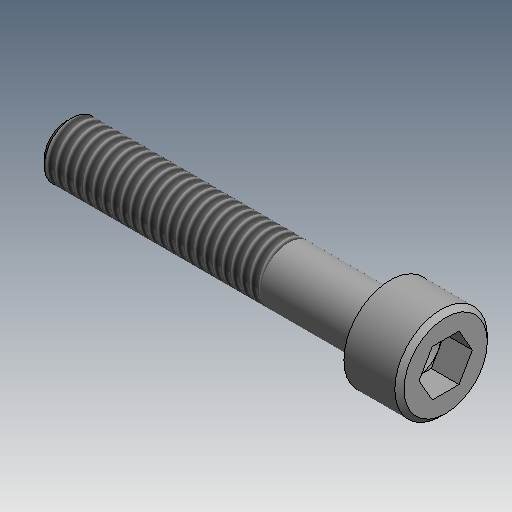
# Autodesk Inventor part: CBM6-35
Saved by Autodesk Inventor 2020 (Build 240168000, 168)
## iProperties
Part Number: CBM6-35
Material: 一般
Catalog Web Link: www.cadenas.de
Description: CBM-Hex Socket Head Cap Screws - Bright Chromate Plating
Vendor: MISUMI
Document SubType Name: Modeling
Designer: partserver
Manufacturer: MISUMI
Mass: 1.3796 g
Surface Area: 10.4152 cm^2
Volume: 1.3796 cm^3
Density: 1 g/cm^3
Appearance: PSOLRGB-192-192-192
Category: PARTsolutions
Company: MISUMI
PSOL_IDENT_0: {$CADENAS_DATA\23d-libs\misumi\metric\27_screws_nuts\cbm.prj},153 {VTYP=3D},{NB=CBM6-35},{LINA=CBM6-
PSOL_IDENT_1: 35},{NN=CBM},{DATE=07.06.2021 12:24:55},{GEOMDATE=24.03.2015 11:44:00},{VERSION=},{LINEID=30},{WBVAR=
PSOL_IDENT_2: L},{WBNUMERIC=L}  {NB=CBM6-35},{LINA=CBM6-35},{KT=DUMMY},{PN=CBM6-35},{TYPE=CBM},{M=6},{M1=6},{L=35}
PSOL_IDENT_3: ,{LALG=8,10,12,14,15,16,18,20,22,25,30,35,40,45,50,60},{LL=24},{A=10.0},{E=6},{B=5.0},{LL3D=24},{TT3
PSOL_IDENT_4: D=3},{R3D=0.250},{C3D=0.5},{A3D=-45}
NB: CBM6-35
NN: CBM
NT: Hex Socket Head Cap Screws - Bright Chromate Plating
NBSYN: $PN.
LINA: CBM6-35
CATALOG: Misumi
PN: CBM6-35
M: 6
L: 35
LL: 24
A: 10
E: 6
B: 5
SUPPLIER: MISUMI
ARTICLENO: CBM6-35
BOMINFO: CBM6-35
CREATOR: CADENAS GmbH
d12: 0.000 mm
d13: 0.000 mm
Title: CBM6-35
Author: Cadenas PARTsolutions
Comments: Hex Socket Head Cap Screws - Bright Chromate Plating
Autodesk Inventor part; units mm, degrees
sketch "Sketch_8" plane through (0, 0, 0) normal (0, 0, 1) x (1, 0, 0)
  line L0 (35, 0) -> (-6, 0)
  line L1 (-6, 0) -> (-6, 4.5)
  line L2 (-6, 4.5) -> (-5.5, 5)
  line L3 (-5.5, 5) -> (0, 5)
  line L4 (0, 5) -> (0, 3.25)
  arc A0 (0, 3.25) -> (0.25, 3) centre (0.25, 3.25) ccw
  line L5 (0.25, 3) -> (34.3865, 3)
  line L6 (34.3865, 3) -> (35, 2.3865)
  line L7 (35, 2.3865) -> (35, 0)
  line L8 (35, 0) -> (-6, 0)
  constraints: 18 end point, 2 point on circle, 1 centre point
revolve "Revolution1" add sketch "Sketch_8" angle 360 about axis through (35, 0, 0) along (1, 0, 0)
thread "Thread1" size "M6x1" class "6g" standard "ISO Metric profile" length 23.3865
sketch "Sketch2" plane through (-6, 0, 0) normal (-1, 0, 0) x (0, 0, 1)
  point P0 (0, 0)
hole "Hole1" at (-6, 0, 0) direction (1, 0, 0) diameter 5 depth 3 tip angle 120
sketch "Sketch_3" plane through (-6, 0, 0) normal (1, 0, 0) x (0, 0, -1)
  line L0 (-2.5, -1.4434) -> (0, -2.8868)
  line L1 (0, -2.8868) -> (2.5, -1.4434)
  line L2 (2.5, -1.4434) -> (2.5, 1.4434)
  line L3 (2.5, 1.4434) -> (0, 2.8868)
  line L4 (0, 2.8868) -> (-2.5, 1.4434)
  line L5 (-2.5, 1.4434) -> (-2.5, -1.4434)
  constraints: 12 end point
extrude "Extrusion1" cut sketch "Sketch_3" along normal blind 3
ref_plane "bolt_XY" through (0, 0, 0) normal (1, 0, 0) x (0, 0, -1)
ref_plane "bolt_YZ" through (0, 0, 0) normal (0, 0, -1) x (0, 1, 0)
ref_plane "bolt_ZX" through (0, 0, 0) normal (0, 1, 0) x (1, 0, 0)
ref_plane "nut_XY" through (35, 0, 0) normal (1, 0, 0) x (0, 0, -1)
ref_plane "nut_YZ" through (35, 0, 0) normal (0, 0, -1) x (0, 1, 0)
ref_plane "nut_ZX" through (35, 0, 0) normal (0, 1, 0) x (1, 0, 0)
body "Solid1"
